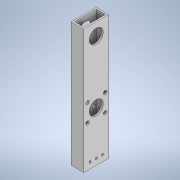
# Autodesk Inventor part: Arm Mount
Saved by Autodesk Inventor 2022 (Build 260153000, 153)
## iProperties
Created: 2023-01-20
Part Number: Arm Mount
Material: Generic
Document SubType Name: Modeling
Designer: s135320
Density: 1 g/cm^3
Appearance: Default
Author: s135320
Autodesk Inventor part; units mm, degrees
ref_plane "YZ Plane" through (0, 0, 0) normal (1, 0, 0) x (0, 1, 0)
ref_plane "XZ Plane" through (0, 0, 0) normal (0, 1, 0) x (-1, 0, 0)
ref_plane "XY Plane" through (0, 0, 0) normal (0, 0, 1) x (1, 0, 0)
sketch "Sketch1" plane through (0, 0, 0) normal (0, 1, 0) x (-1, 0, 0)
  line L0 (0, 0) -> (25.4, 0)
  line L1 (25.4, 0) -> (25.4, -50.8)
  line L2 (25.4, -50.8) -> (0, -50.8)
  line L3 (0, -50.8) -> (0, 0)
  dimension "d0" = 25.4
  dimension "d1" = 50.8
  constraints: 8 end point, 2 parallel, 1 horizontal, 1 perpendicular
  measures "d0" distance of L1.end L2.end
  measures "d1" distance of L0.end L1.end
extrude "Extrusion1" add sketch "Sketch1" along normal blind 254
shell "Shell1" thickness 3.175 removed faces 2 at (-8.4667, 254, -33.8667) at (-8.4667, 0, -33.8667)
sketch "Sketch2" plane through (0, 0, 0) normal (1, 0, 0) x (0, 0, -1)
  line L0 (0, 0) -> (0, 254) projected
  line L1 (0, 12.7) -> (50.8, 12.7)
  line L2 (50.8, 0) -> (50.8, 254) projected
  circle A0 centre (25.4, 12.7) radius 2.0701
  circle A1 centre (38.1, 12.7) radius 2.0701
  circle A2 centre (12.7, 12.7) radius 2.0701
  line L3 (0, 0) -> (50.8, 0) projected
  line L4 (3.175, 254) -> (47.625, 254) projected
  line L5 (25.4, 254) -> (25.4, 228.6)
  circle A3 centre (25.4, 228.6) radius 14.2875
  line L6 (25.4, 228.6) -> (25.4, 102.1842)
  circle A4 centre (25.4, 102.1842) radius 14.2875
  circle A5 centre (25.4, 102.1842) radius 25.4 construction
  line L7 (25.4, 102.1842) -> (43.3605, 120.1447) construction
  line L8 (25.4, 102.1842) -> (50.8, 102.1842) construction
  line L9 (25.4, 102.1842) -> (43.3605, 84.2237) construction
  line L10 (25.4, 102.1842) -> (7.4395, 84.2237) construction
  line L11 (25.4, 102.1842) -> (7.4395, 120.1447) construction
  circle A6 centre (7.4395, 120.1447) radius 3.4925
  circle A7 centre (43.3605, 120.1447) radius 3.4925
  circle A8 centre (43.3605, 84.2237) radius 3.4925
  circle A9 centre (7.4395, 84.2237) radius 3.4925
  dimension "d5" = 4.1402
  dimension "d8" = 12.7
  dimension "d15" = 12.7
  dimension "d22" = 12.7
  dimension "d23" = 25.4
  dimension "d24" = 28.575
  dimension "d25" = 28.575
  dimension "d26" = 126.4158
  dimension "d27" = 50.8
  dimension "d28" = 45
  dimension "d29" = 6.985
  dimension "d30" = 6.985
  dimension "d31" = 6.985
  dimension "d32" = 6.985
  constraints: 16 end point, 10 centre point, 7 coincident, 4 horizontal, 4 point on circle, 3 point on line, 2 midpoint, 2 vertical, 1 equal length, 1 perpendicular, 4 other
  measures "d5" diameter of A0
  measures "d8" distance of A0.centre A1.centre
  measures "d15" distance of A0.centre A2.centre
  measures "d22" distance between parallel lines of L3 L1
  measures "d23" distance of L5.start L5.end
  measures "d24" diameter of A3
  measures "d25" diameter of A4
  measures "d26" distance of L6.end L5.end
  measures "d27" diameter of A5
  measures "d28" angle of L8 L7
  measures "d29" diameter of A6
  measures "d30" diameter of A7
  measures "d31" diameter of A8
  measures "d32" diameter of A9
extrude "Extrusion2" cut sketch "Sketch2" against normal through all contours A2 L1 | L1 A2 | A1 L1 | L1 A1 | A0 L1 | L1 A0 | A3 L6 L5 | L5 L6 A3 | A4 | A6 | A7 | A8 | A9
body "Solid1"
